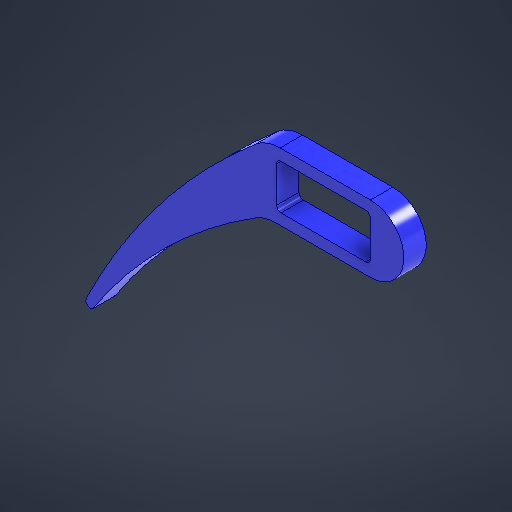
# Autodesk Inventor part: Spider_Robot_Tibia_V1
Saved by Autodesk Inventor 2026.2 (Build 302298010, 298A)
## iProperties
Created: 2026-08-14
Part Number: Spider_Robot_Tibia_V1
Material: Generic
Document SubType Name: Modeling
Designer: Entity
Mass: 24.8327 g
Surface Area: 100.14 cm^2
Volume: 24.8327 cm^3
Density: 1 g/cm^3
Appearance: Blue - Wall Paint - Glossy
Author: Entity
Autodesk Inventor part; units mm, degrees
ref_plane "YZ Plane" through (0, 0, 0) normal (1, 0, 0) x (0, 1, 0)
ref_plane "XZ Plane" through (0, 0, 0) normal (0, 1, 0) x (-1, 0, 0)
ref_plane "XY Plane" through (0, 0, 0) normal (0, 0, 1) x (1, 0, 0)
sketch "Sketch1" plane through (0, 0, 0) normal (0, 0, 1) x (1, 0, 0)
  line L0 (-21, 10) -> (21, 10)
  line L1 (21, 10) -> (21, -10)
  line L2 (21, -10) -> (-21, -10)
  line L3 (-21, -10) -> (-21, 10)
  arc A0 (21, -15) -> (36, 0) centre (21, 0) ccw
  arc A1 (21, -15) -> (21, 15) centre (21, 0) ccw
  line L4 (21, 15) -> (-19.3814, 15)
  line L5 (21, -15) -> (-21.3289, -15)
  arc A2 (-30.3889, 10.9551) -> (-106.2021, -86.7378) centre (164.8345, -218.8085) ccw
  arc A3 (-106.2021, -86.7378) -> (-103.2462, -89.2462) centre (-104.4035, -87.6142) ccw
  arc A4 (-30.3302, -17.5786) -> (-103.2462, -89.2462) centre (94.391, -217.3993) ccw
  arc A5 (-19.3814, 15) -> (-30.3889, 10.9551) centre (-19.3814, -2) ccw
  arc A6 (-21.3289, -15) -> (-30.3302, -17.5786) centre (-21.3289, -32) ccw
  point P0 (0, 0)
  point P1 (-21, 0)
  point P2 (-26.1005, -15)
  point P3 (-25.5259, 15)
  dimension "d0" = 42
  dimension "d1" = 20
  dimension "d2" = 10
  dimension "d3" = 21
  dimension "d5" = 15
  dimension "d15" = 301.502
  dimension "d16" = 235.5497
  dimension "d17" = 17
  constraints: 17 point on circle, 12 end point, 7 centre point, 5 tangent, 3 horizontal, 2 parallel, 2 point on line, 1 equal radius, 1 midpoint, 1 perpendicular
  measures "d0" distance of L0.start L0.end
  measures "d1" distance of L2.end L0.start
  measures "d2" distance from line of L0 point (0, 0)
  measures "d3" distance of point (-21, 0) point (0, 0)
  measures "d5" radius of A1
  measures "d15" radius of A2
  measures "d16" radius of A4
  measures "d17" radius of A5
extrude "Extrusion1" add sketch "Sketch1" along normal blind 10
fillet "Fillet1" radius 2 4 edges at (21, 10, 5) (21, -10, 5) (-21, 10, 5) (-21, -10, 5)
body "Solid1"
